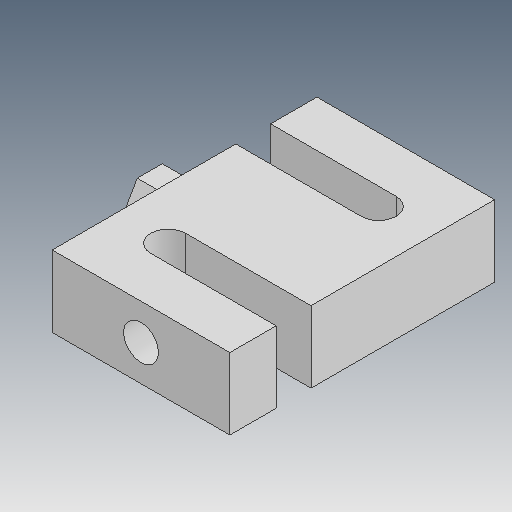
# Autodesk Inventor part: tension_sensor
Saved by Autodesk Inventor 2025.2 (Build 292293000, 293)
## iProperties
Created: 2025-02-16
Part Number: tension_sensor
Material: Generic
Document SubType Name: Modeling
Designer: email
Density: 1 g/cm^3
Appearance: Default
Author: email
Autodesk Inventor part; units mm, degrees
ref_plane "YZ Plane" through (0, 0, 0) normal (1, 0, 0) x (0, 1, 0)
ref_plane "XZ Plane" through (0, 0, 0) normal (0, 1, 0) x (-1, 0, 0)
ref_plane "XY Plane" through (0, 0, 0) normal (0, 0, 1) x (1, 0, 0)
sketch "Sketch1" plane through (0, 0, 0) normal (0, 1, 0) x (-1, 0, 0)
  line L0 (0, 0) -> (0, -52.7)
  line L1 (0, -52.7) -> (-36, -52.7)
  arc A0 (-36, -52.7) -> (-36, -62.7) centre (-36, -57.7) ccw
  line L2 (-36, -62.7) -> (0, -62.7)
  line L3 (0, -62.7) -> (0, -76)
  line L4 (0, -76) -> (-51, -76)
  line L5 (-51, -76) -> (-51, -23.3)
  line L6 (-51, -23.3) -> (-15, -23.3)
  arc A1 (-15, -23.3) -> (-15, -13.3) centre (-15, -18.3) ccw
  line L7 (-15, -13.3) -> (-51, -13.3)
  line L8 (-51, -13.3) -> (-51, 0)
  line L9 (-51, 0) -> (0, 0)
  point P0 (-25.5, -76)
  dimension "d0" = 76
  dimension "d1" = 10
  dimension "d2" = 10
  dimension "d3" = 29.4
  dimension "d4" = 13.3
  dimension "d17" = 51
  dimension "d18" = 15
  dimension "d19" = 15
  constraints: 20 end point, 6 perpendicular, 5 point on circle, 4 tangent, 2 centre point, 2 collinear, 2 vertical, 1 horizontal, 1 midpoint, 1 parallel
  measures "d0" distance from line of L9 point (-25.5, -76)
  measures "d1" distance between parallel lines of L1 L2
  measures "d2" distance between parallel lines of L7 L6
  measures "d3" distance between parallel lines of L6 L1
  measures "d4" distance between parallel lines of L4 L2
  measures "d17" distance between parallel lines of L5 L0
  measures "d18" distance from line of L5 A0.centre
  measures "d19" distance from line of L0 A1.centre
extrude "Extrusion1" add sketch "Sketch1" along normal blind 20.5
sketch "Sketch2" plane through (0, 0, 0) normal (0, 0, 1) x (1, 0, 0)
  circle A0 centre (25.5, 10.25) radius 5
  line L0 (0, 0) -> (51, 0) projected
  line L1 (0, 0) -> (0, 20.5) projected
  point P0 (25.5, 0)
  point P1 (0, 10.25)
  dimension "d7" = 10
  constraints: 2 midpoint, 1 centre point, 1 horizontal alignment, 1 vertical alignment
  measures "d7" diameter of A0
extrude "Extrusion2" cut sketch "Sketch2" against normal up to next
sketch "Sketch3" plane through (51, 0, -76) normal (0, 0, -1) x (-1, 0, 0)
  circle A0 centre (25.5, 10.25) radius 5 projected
  circle A1 centre (25.5, 10.25) radius 5
  point P0 (51, 0)
  point P1 (31.0896, 7.7494)
  point P2 (31.0896, 12.7506)
  point P3 (30.0641, 8.2082)
  point P4 (30.0641, 12.2918)
  dimension "d10" = 5
  constraints: 1 centre point, 1 coincident, 1 other
extrude "Extrusion3" cut sketch "Sketch3" against normal blind 10
sketch "Sketch4" plane through (0, 0, -52.7) normal (-1, 0, 0) x (0, 0, 1)
  line L0 (21.8591, 9.9441) -> (18.2796, 3.7441)
  line L1 (18.2796, 3.7441) -> (11.1204, 3.7441)
  line L2 (11.1204, 3.7441) -> (7.5409, 9.9441)
  line L3 (7.5409, 9.9441) -> (11.1204, 16.1441)
  line L4 (11.1204, 16.1441) -> (18.2796, 16.1441)
  line L5 (18.2796, 16.1441) -> (21.8591, 9.9441)
  line L6 (-23.3, 0) -> (-23.3, 20.5) projected
  point P0 (52.7, 0)
  point P1 (14.7, 9.9441)
  point P2 (-23.3, 10.25)
  dimension "d13" = 12.4
  dimension "d14" = 38
  constraints: 12 end point, 1 horizontal, 1 midpoint, 13 other
  measures "d13" distance between parallel lines of L5 L2
  measures "d14" horizontal distance of point (-23.3, 10.25) point (14.7, 9.944)
extrude "Extrusion4" add sketch "Sketch4" along normal blind 10
body "Solid1"
